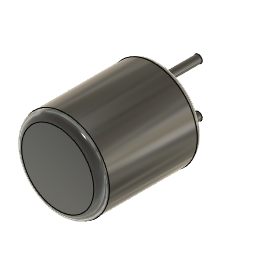
capacitor (Autodesk Fusion 360 design; units mm, degrees)
Autodesk Fusion 360 part; units mm, degrees
sketch "Sketch1" plane through (0, 0, 0) normal (0, 1, 0) x (1, 0, 0)
  circle A0 centre (0, 0) radius 2.25
  dimension "d1" = 4.5
  constraint coincident A0.centre origin
  measures "d1" diameter of A0
extrude "Extrude1" add sketch "Sketch1" along normal blind 5.2
sketch "Sketch2" plane through (0, 5.2, 0) normal (0, 1, 0) x (-1, 0, 0)
  circle A0 centre (0, 0) radius 2.25
  line L0 (0, 0) -> (0, -1.27)
  circle A1 centre (0, -1.27) radius 0.2
  line L1 (0, 0) -> (-0.6583, 0) construction
  circle A2 centre (0, 1.27) radius 0.2
  dimension "d4" = 1.27
  dimension "d6" = 0.4
  constraint coincident A0.centre L0.start
  constraint vertical L0
  constraint coincident L0.end A1.centre
  constraint symmetric A1 L1 A2
  measures "d4" distance of A0.centre L0.end
  measures "d6" diameter of A1
extrude "Extrude2" add sketch "Sketch2" along normal blind 2 contours A1 | A2
fillet "Fillet1" radius 0.4 1 edges at (-2.0977, 0, 0.8136)
fillet "Fillet2" radius 0.3 1 edges at (-2.0977, 5.2, 0.8136)
sketch "Sketch3" plane through (0, 0, 0) normal (0, 0, 1) x (1, 0, 0)
equation "d4 = ( 2.54 / 2 ) * 1 mm"
